Autodesk Fusion 360 part; units mm, degrees
(part 2 of 2)
sketch "スケッチ3" plane through (0, 0, 1.5) normal (0, 0, 1) x (-1, 0, 0)
  line L0 (-5.6421, -16.3724) -> (-10.7928, -25.2936)
  arc A0 (-10.7928, -25.2936) -> (-3.3, -27.3013) centre (0, 0) ccw
  line L1 (-3.3, -27.3013) -> (-3.3, -17)
  line L2 (-3.3, -17) -> (3.3, -17)
  line L3 (3.3, -17) -> (3.3, -27.3013)
  arc A1 (3.3, -27.3013) -> (10.7928, -25.2936) centre (0, 0) ccw
  line L4 (10.7928, -25.2936) -> (5.6421, -16.3724)
  line L5 (5.6421, -16.3724) -> (11.3579, -13.0724)
  line L6 (11.3579, -13.0724) -> (16.5085, -21.9936)
  arc A2 (16.5085, -21.9936) -> (21.9936, -16.5085) centre (0, 0) ccw
  line L7 (21.9936, -16.5085) -> (13.0724, -11.3579)
  line L8 (13.0724, -11.3579) -> (16.3724, -5.6421)
  line L9 (16.3724, -5.6421) -> (25.2936, -10.7928)
  arc A3 (25.2936, -10.7928) -> (27.3013, -3.3) centre (0, 0) ccw
  line L10 (27.3013, -3.3) -> (17, -3.3)
  line L11 (17, -3.3) -> (17, 3.3)
  line L12 (17, 3.3) -> (27.3013, 3.3)
  arc A4 (27.3013, 3.3) -> (25.2936, 10.7928) centre (0, 0) ccw
  line L13 (25.2936, 10.7928) -> (16.3724, 5.6421)
  line L14 (16.3724, 5.6421) -> (13.0724, 11.3579)
  line L15 (13.0724, 11.3579) -> (21.9936, 16.5085)
  arc A5 (21.9936, 16.5085) -> (16.5085, 21.9936) centre (0, 0) ccw
  line L16 (16.5085, 21.9936) -> (11.3579, 13.0724)
  line L17 (11.3579, 13.0724) -> (5.6421, 16.3724)
  line L18 (5.6421, 16.3724) -> (10.7928, 25.2936)
  arc A6 (10.7928, 25.2936) -> (3.3, 27.3013) centre (0, 0) ccw
  line L19 (3.3, 27.3013) -> (3.3, 17)
  line L20 (3.3, 17) -> (-3.3, 17)
  line L21 (-3.3, 17) -> (-3.3, 27.3013)
  arc A7 (-3.3, 27.3013) -> (-10.7928, 25.2936) centre (0, 0) ccw
  line L22 (-10.7928, 25.2936) -> (-5.6421, 16.3724)
  line L23 (-5.6421, 16.3724) -> (-11.3579, 13.0724)
  line L24 (-11.3579, 13.0724) -> (-16.5085, 21.9936)
  arc A8 (-16.5085, 21.9936) -> (-21.9936, 16.5085) centre (0, 0) ccw
  line L25 (-21.9936, 16.5085) -> (-13.0724, 11.3579)
  line L26 (-13.0724, 11.3579) -> (-16.3724, 5.6421)
  line L27 (-16.3724, 5.6421) -> (-25.2936, 10.7928)
  arc A9 (-25.2936, 10.7928) -> (-27.3013, 3.3) centre (0, 0) ccw
  line L28 (-27.3013, 3.3) -> (-17, 3.3)
  line L29 (-17, 3.3) -> (-17, -3.3)
  line L30 (-17, -3.3) -> (-27.3013, -3.3)
  arc A10 (-27.3013, -3.3) -> (-25.2936, -10.7928) centre (0, 0) ccw
  line L31 (-25.2936, -10.7928) -> (-16.3724, -5.6421)
  line L32 (-16.3724, -5.6421) -> (-13.0724, -11.3579)
  line L33 (-13.0724, -11.3579) -> (-21.9936, -16.5085)
  arc A11 (-21.9936, -16.5085) -> (-16.5085, -21.9936) centre (0, 0) ccw
  line L34 (-16.5085, -21.9936) -> (-11.3579, -13.0724)
  line L35 (-11.3579, -13.0724) -> (-5.6421, -16.3724)
  line L36 (3.3, -27.3013) -> (3.3, -26.1013)
  line L37 (3.3, -26.1013) -> (3.3, -23.5013)
  line L38 (3.3, -23.5013) -> (5.3, -23.5013)
  line L39 (5.3, -23.5013) -> (5.3, -26.1013)
  line L40 (5.3, -26.1013) -> (3.3, -26.1013)
  line L41 (3.3, -26.1013) -> (3.3, -23.5013)
  line L42 (-3.3, -27.3013) -> (-3.3, -26.1013)
  line L43 (-3.3, -26.1013) -> (-5.3, -26.1013)
  line L44 (-5.3, -26.1013) -> (-5.3, -23.5013)
  line L45 (-5.3, -23.5013) -> (-3.3, -23.5013)
  line L46 (-3.3, -23.5013) -> (-3.3, -26.1013)
  line L47 (14.6085, -18.7027) -> (16.3406, -17.7027)
  line L48 (16.3406, -17.7027) -> (17.6406, -19.9544)
  line L49 (17.6406, -19.9544) -> (15.9085, -20.9544)
  line L50 (15.9085, -20.9544) -> (14.6085, -18.7027)
  line L51 (8.8928, -22.0027) -> (10.1928, -24.2544)
  line L52 (7.1607, -23.0027) -> (8.8928, -22.0027)
  line L53 (8.4607, -25.2544) -> (7.1607, -23.0027)
  line L54 (10.1928, -24.2544) -> (8.4607, -25.2544)
  line L55 (22.0027, -8.8928) -> (23.0027, -7.1607)
  line L56 (23.0027, -7.1607) -> (25.2544, -8.4607)
  line L57 (25.2544, -8.4607) -> (24.2544, -10.1928)
  line L58 (24.2544, -10.1928) -> (22.0027, -8.8928)
  line L59 (18.7027, -14.6085) -> (20.9544, -15.9085)
  line L60 (17.7027, -16.3406) -> (18.7027, -14.6085)
  line L61 (19.9544, -17.6406) -> (17.7027, -16.3406)
  line L62 (20.9544, -15.9085) -> (19.9544, -17.6406)
  line L63 (23.5013, 3.3) -> (23.5013, 5.3)
  line L64 (23.5013, 5.3) -> (26.1013, 5.3)
  line L65 (26.1013, 5.3) -> (26.1013, 3.3)
  line L66 (26.1013, 3.3) -> (23.5013, 3.3)
  line L67 (23.5013, -3.3) -> (26.1013, -3.3)
  line L68 (23.5013, -5.3) -> (23.5013, -3.3)
  line L69 (26.1013, -5.3) -> (23.5013, -5.3)
  line L70 (26.1013, -3.3) -> (26.1013, -5.3)
  line L71 (18.7027, 14.6085) -> (17.7027, 16.3406)
  line L72 (17.7027, 16.3406) -> (19.9544, 17.6406)
  line L73 (19.9544, 17.6406) -> (20.9544, 15.9085)
  line L74 (20.9544, 15.9085) -> (18.7027, 14.6085)
  line L75 (22.0027, 8.8928) -> (24.2544, 10.1928)
  line L76 (23.0027, 7.1607) -> (22.0027, 8.8928)
  line L77 (25.2544, 8.4607) -> (23.0027, 7.1607)
  line L78 (24.2544, 10.1928) -> (25.2544, 8.4607)
  line L79 (8.8928, 22.0027) -> (7.1607, 23.0027)
  line L80 (7.1607, 23.0027) -> (8.4607, 25.2544)
  line L81 (8.4607, 25.2544) -> (10.1928, 24.2544)
  line L82 (10.1928, 24.2544) -> (8.8928, 22.0027)
  line L83 (14.6085, 18.7027) -> (15.9085, 20.9544)
  line L84 (16.3406, 17.7027) -> (14.6085, 18.7027)
  line L85 (17.6406, 19.9544) -> (16.3406, 17.7027)
  line L86 (15.9085, 20.9544) -> (17.6406, 19.9544)
  line L87 (-3.3, 23.5013) -> (-5.3, 23.5013)
  line L88 (-5.3, 23.5013) -> (-5.3, 26.1013)
  line L89 (-5.3, 26.1013) -> (-3.3, 26.1013)
  line L90 (-3.3, 26.1013) -> (-3.3, 23.5013)
  line L91 (3.3, 23.5013) -> (3.3, 26.1013)
  line L92 (5.3, 23.5013) -> (3.3, 23.5013)
  line L93 (5.3, 26.1013) -> (5.3, 23.5013)
  line L94 (3.3, 26.1013) -> (5.3, 26.1013)
  line L95 (-14.6085, 18.7027) -> (-16.3406, 17.7027)
  line L96 (-16.3406, 17.7027) -> (-17.6406, 19.9544)
  line L97 (-17.6406, 19.9544) -> (-15.9085, 20.9544)
  line L98 (-15.9085, 20.9544) -> (-14.6085, 18.7027)
  line L99 (-8.8928, 22.0027) -> (-10.1928, 24.2544)
  line L100 (-7.1607, 23.0027) -> (-8.8928, 22.0027)
  line L101 (-8.4607, 25.2544) -> (-7.1607, 23.0027)
  line L102 (-10.1928, 24.2544) -> (-8.4607, 25.2544)
  line L103 (-22.0027, 8.8928) -> (-23.0027, 7.1607)
  line L104 (-23.0027, 7.1607) -> (-25.2544, 8.4607)
  line L105 (-25.2544, 8.4607) -> (-24.2544, 10.1928)
  line L106 (-24.2544, 10.1928) -> (-22.0027, 8.8928)
  line L107 (-18.7027, 14.6085) -> (-20.9544, 15.9085)
  line L108 (-17.7027, 16.3406) -> (-18.7027, 14.6085)
  line L109 (-19.9544, 17.6406) -> (-17.7027, 16.3406)
  line L110 (-20.9544, 15.9085) -> (-19.9544, 17.6406)
  line L111 (-23.5013, -3.3) -> (-23.5013, -5.3)
  line L112 (-23.5013, -5.3) -> (-26.1013, -5.3)
  line L113 (-26.1013, -5.3) -> (-26.1013, -3.3)
  line L114 (-26.1013, -3.3) -> (-23.5013, -3.3)
  line L115 (-23.5013, 3.3) -> (-26.1013, 3.3)
  line L116 (-23.5013, 5.3) -> (-23.5013, 3.3)
  line L117 (-26.1013, 5.3) -> (-23.5013, 5.3)
  line L118 (-26.1013, 3.3) -> (-26.1013, 5.3)
  line L119 (-18.7027, -14.6085) -> (-17.7027, -16.3406)
  line L120 (-17.7027, -16.3406) -> (-19.9544, -17.6406)
  line L121 (-19.9544, -17.6406) -> (-20.9544, -15.9085)
  line L122 (-20.9544, -15.9085) -> (-18.7027, -14.6085)
  line L123 (-22.0027, -8.8928) -> (-24.2544, -10.1928)
  line L124 (-23.0027, -7.1607) -> (-22.0027, -8.8928)
  line L125 (-25.2544, -8.4607) -> (-23.0027, -7.1607)
  line L126 (-24.2544, -10.1928) -> (-25.2544, -8.4607)
  line L127 (-8.8928, -22.0027) -> (-7.1607, -23.0027)
  line L128 (-7.1607, -23.0027) -> (-8.4607, -25.2544)
  line L129 (-8.4607, -25.2544) -> (-10.1928, -24.2544)
  line L130 (-10.1928, -24.2544) -> (-8.8928, -22.0027)
  line L131 (-14.6085, -18.7027) -> (-15.9085, -20.9544)
  line L132 (-16.3406, -17.7027) -> (-14.6085, -18.7027)
  line L133 (-17.6406, -19.9544) -> (-16.3406, -17.7027)
  line L134 (-15.9085, -20.9544) -> (-17.6406, -19.9544)
  circle A12 centre (0, -6.25) radius 1.65
  circle A13 centre (5.4127, 3.125) radius 1.65
  circle A14 centre (-5.4127, 3.125) radius 1.65
  line L135 (4.752, 5.6303) -> (0, 2.8868)
  line L136 (0, 2.8868) -> (-4.752, 5.6303)
  line L137 (-4.752, 5.6303) -> (-6.2309, 14.1924)
  arc A15 (6.2309, 14.1924) -> (-6.2309, 14.1924) centre (0, 0) ccw
  line L138 (6.2309, 14.1924) -> (4.752, 5.6303)
  circle A16 centre (0, 0) radius 2.1
  arc A17 (15.4284, 1.4885) -> (9.0033, 12.6171) centre (0, 0) ccw
  line L139 (15.4284, 1.4885) -> (7.5798, 4.3762)
  line L140 (7.5798, 4.3762) -> (9.0033, 12.6171)
  line L141 (2.5, -6.9305) -> (2.5, -1.4434)
  line L142 (2.5, -1.4434) -> (7.252, 1.3002)
  line L143 (7.252, 1.3002) -> (15.4065, -1.7001)
  arc A18 (9.1755, -12.4924) -> (15.4065, -1.7001) centre (0, 0) ccw
  line L144 (9.1755, -12.4924) -> (2.5, -6.9305)
  arc A19 (-9.0033, 12.6171) -> (-15.4284, 1.4885) centre (0, 0) ccw
  line L145 (-9.0033, 12.6171) -> (-7.5798, 4.3762)
  line L146 (-7.5798, 4.3762) -> (-15.4284, 1.4885)
  line L147 (-6.4251, -14.1056) -> (0, -8.7524)
  line L148 (0, -8.7524) -> (6.4251, -14.1056)
  arc A20 (-6.4251, -14.1056) -> (6.4251, -14.1056) centre (0, 0) ccw
  line L149 (-2.5, -6.9305) -> (-9.1755, -12.4924)
  arc A21 (-15.4065, -1.7001) -> (-9.1755, -12.4924) centre (0, 0) ccw
  line L150 (-15.4065, -1.7001) -> (-7.252, 1.3002)
  line L151 (-7.252, 1.3002) -> (-2.5, -1.4434)
  line L152 (-2.5, -1.4434) -> (-2.5, -6.9305)
  dimension "d32" = 1.2
  dimension "d33" = 2.6
  dimension "d34" = 2
  dimension "d35" = 2.6
  dimension "d36" = 1.2
  dimension "d37" = 2
  dimension "d38" = 2.6
  dimension "d40" = 360
  constraint coincident L3.end A1.start
  constraint vertical L36
  constraint parallel L3 L37
  constraint horizontal L38
  constraint vertical L39
  constraint horizontal L40
  constraint vertical L41
  constraint coincident A0.end L1.start
  constraint parallel L1 L42
  constraint horizontal L43
  constraint vertical L44
  constraint horizontal L45
  constraint vertical L46
  measures "d32" distance of L3.end L36.end
  measures "d33" distance of L36.end L37.end
  measures "d34" distance of L37.end L38.end
  measures "d35" distance of L37.end L36.end
  measures "d36" distance of A0.end L42.end
  measures "d37" distance of L42.end L43.end
  measures "d38" distance of L42.end L45.end
extrude "押し出し3" add sketch "スケッチ3" along normal blind 0.5 contours L0 A0 L1 L2 L3 A1 L4 L5 L6 A2 L7 L8 L9 A3 L10 L11 L12 A4 L13 L14 L15 A5 L16 L17 L18 A6 L19 L20 L21 A7 L22 L23 L24 A8 L25 L26 L27 A9 L28 L29 L30 A10 L31 L32 L33 A11 L34 L35 L36 L38 L39 L40 L42 L43 L44 L45 L47 L48 L49 L52 L53 L54 L55 L56 L57 L60 L61 L62 L63 L64 L65 L68 L69 L70 L71 L72 L73 L76 L77 L78 L79 L80 L81 L84 L85 L86 L87 L88 L89 L92 L93 L94 L95 L96 L97 L100 L101 L102 L103 L104 L105 L108 L109 L110 L111 L112 L113 L116 L117 L118 L119 L120 L121 L124 L125 L126 L127 L128 L129 L132 L133 L134
extrude "押し出し4" cut 1 faces at (12.6956, -0.3629, 0) along direction (0, 0, 1) blind 0.5
fillet "フィレット1" radius 1.5 10 edges at (-9.1755, 12.4924, 1.25) (0, -2.8868, 1.25) (-2.5, 1.4434, 1.25) (-2.5, 6.9305, 1.25) (0, 8.7524, 1.25) (-6.4251, 14.1056, 1.25) (6.4251, 14.1056, 1.25) (9.1755, 12.4924, 1.25) (2.5, 6.9305, 1.25) (2.5, 1.4434, 1.25)
fillet "フィレット1" radius 1.5 14 edges at (-4.752, -5.6303, 1.25) (-7.5798, -4.3762, 1.25) (-7.252, -1.3002, 1.25) (-15.4284, -1.4885, 1.25) (-15.4065, 1.7001, 1.25) (-6.2309, -14.1924, 1.25) (-9.0033, -12.6171, 1.25) (6.2309, -14.1924, 1.25) (9.0033, -12.6171, 1.25) (4.752, -5.6303, 1.25) (15.4284, -1.4885, 1.25) (7.5798, -4.3762, 1.25) (7.252, -1.3002, 1.25) (15.4065, 1.7001, 1.25)
fillet "フィレット2" radius 0.5 4 edges at (17.7027, 16.3406, 1.75) (19.9544, 17.6406, 1.75) (23.0027, 7.1607, 1.75) (25.2544, 8.4607, 1.75)
fillet "フィレット3" radius 0.5 44 edges at (17.6406, 19.9544, 1.75) (16.3406, 17.7027, 1.75) (8.4607, 25.2544, 1.75) (5.3, 23.5013, 1.75) (7.1607, 23.0027, 1.75) (5.3, 26.1013, 1.75) (-5.3, 23.5013, 1.75) (-5.3, 26.1013, 1.75) (-8.4607, 25.2544, 1.75) (-7.1607, 23.0027, 1.75) (-17.6406, 19.9544, 1.75) (-16.3406, 17.7027, 1.75) (-19.9544, 17.6406, 1.75) (-17.7027, 16.3406, 1.75) (-25.2544, 8.4607, 1.75) (-23.0027, 7.1607, 1.75) (-23.5013, 5.3, 1.75) (-26.1013, 5.3, 1.75) (-26.1013, -5.3, 1.75) (-23.5013, -5.3, 1.75) (-23.0027, -7.1607, 1.75) (-25.2544, -8.4607, 1.75) (-17.7027, -16.3406, 1.75) (-16.3406, -17.7027, 1.75) (-19.9544, -17.6406, 1.75) (-17.6406, -19.9544, 1.75) (-7.1607, -23.0027, 1.75) (-5.3, -23.5013, 1.75) (-5.3, -26.1013, 1.75) (-8.4607, -25.2544, 1.75) (7.1607, -23.0027, 1.75) (5.3, -23.5013, 1.75) (8.4607, -25.2544, 1.75) (5.3, -26.1013, 1.75) (16.3406, -17.7027, 1.75) (17.7027, -16.3406, 1.75) (19.9544, -17.6406, 1.75) (17.6406, -19.9544, 1.75) (23.5013, -5.3, 1.75) (23.0027, -7.1607, 1.75) (25.2544, -8.4607, 1.75) (26.1013, -5.3, 1.75) (26.1013, 5.3, 1.75) (23.5013, 5.3, 1.75)
fillet "フィレット4" radius 1.5 24 edges at (13.0724, 11.3579, 1.25) (11.3579, 13.0724, 1.25) (5.6421, 16.3724, 1.25) (3.3, 17, 1.25) (-3.3, 17, 1.25) (-5.6421, 16.3724, 1.25) (-11.3579, 13.0724, 1.25) (-13.0724, 11.3579, 1.25) (-16.3724, 5.6421, 1.25) (-17, 3.3, 1.25) (-17, -3.3, 1.25) (-16.3724, -5.6421, 1.25) (-13.0724, -11.3579, 1.25) (-11.3579, -13.0724, 1.25) (-5.6421, -16.3724, 1.25) (-3.3, -17, 1.25) (3.3, -17, 1.25) (5.6421, -16.3724, 1.25) (13.0724, -11.3579, 1.25) (11.3579, -13.0724, 1.25) (17, -3.3, 1.25) (16.3724, -5.6421, 1.25) (17, 3.3, 1.25) (16.3724, 5.6421, 1.25)
extrude "押し出し5" add 1 faces at (6.483, -9.7763, 2) along direction (0, 0, 1) blind 2
extrude "押し出し6" cut 1 faces at (6.483, -9.7763, 4) along direction (0, 0, -1) blind 2

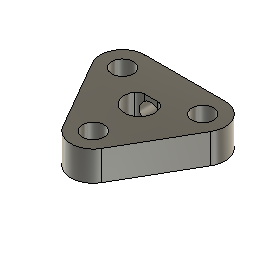
design "オムニ固定"
Autodesk Fusion 360 part; units mm, degrees
sketch "スケッチ1" plane through (0, 0, 0) normal (0, 0, 1) x (1, 0, 0)
  line L0 (2.5981, -7.75) -> (8.0107, 1.625)
  line L1 (0, -6.25) -> (5.4127, 3.125)
  circle A0 centre (5.4127, 3.125) radius 3
  line L2 (5.4127, 3.125) -> (8.0107, 1.625)
  line L3 (5.4127, 3.125) -> (5.4127, 6.125)
  line L4 (5.4127, 3.125) -> (-5.4127, 3.125)
  line L5 (-5.4127, 6.125) -> (5.4127, 6.125)
  circle A1 centre (-5.4127, 3.125) radius 3
  line L6 (-5.4127, 3.125) -> (0, -6.25)
  line L7 (-8.0107, 1.625) -> (-2.5981, -7.75)
  circle A2 centre (0, -6.25) radius 3
  line L8 (0, -6.25) -> (-2.5981, -7.75)
  line L9 (0, -6.25) -> (2.5981, -7.75)
  line L10 (-5.4127, 3.125) -> (-8.0107, 1.625)
  line L11 (-5.4127, 3.125) -> (-5.4127, 6.125)
  circle A3 centre (5.4127, 3.125) radius 1.45
  circle A4 centre (0, 0) radius 2.05
  circle A5 centre (0, -6.25) radius 1.45
  circle A6 centre (-5.4127, 3.125) radius 1.45
  line L12 (0, 0) -> (0, 1.53)
  line L13 (0, 1.53) -> (1.3644, 1.53)
  line L14 (0, 1.53) -> (-1.3644, 1.53)
  dimension "d1" = 6
  dimension "d2" = 6
  dimension "d3" = 6
  dimension "d4" = 2.9
  dimension "d5" = 4.1
  dimension "d6" = 2.9
  dimension "d9" = 2.9
  dimension "d13" = 1.53
  constraint coincident L1.start L6.end
  constraint coincident L1.end A0.centre
  constraint coincident L3.end A0
  constraint vertical L3
  constraint coincident L5.start A1
  constraint perpendicular L4 L11
  constraint coincident L0.end A0
  constraint perpendicular L1 L2
  constraint coincident L0.start A2
  constraint perpendicular L1 L9
  constraint coincident L7.end A2
  constraint perpendicular L6 L8
  constraint coincident L4.end A1.centre
  constraint coincident L7.start A1
  constraint parallel L8 L10
  constraint coincident A4.centre L12.start
  constraint concentric A2 A5
  constraint concentric A1 A6
  constraint vertical L12
  constraint coincident A4 L13.end
  constraint perpendicular L12 L13
  constraint coincident A4 L14.end
  constraint perpendicular L12 L14
  measures "d1" diameter of A2
  measures "d2" diameter of A0
  measures "d3" diameter of A1
  measures "d4" diameter of A3
  measures "d5" diameter of A4
  measures "d6" diameter of A5
  measures "d9" diameter of A6
  measures "d13" distance of A4.centre L12.end
extrude "押し出し1" add sketch "スケッチ1" along normal blind 4 contours L0 L1 A0 A2 | L1 A2 L9 A5 | A2 L8 L9 A5 | A0 L2 L3 A3 | L1 A0 L2 A3 | A1 L6 L7 A2 | L6 A2 L8 A5 | L1 A0 L4 A3 | L1 A0 L4 A1 L6 A2 | A1 L6 L10 A6 | A1 L10 L11 A6 | L1 L6 A2 A5 | A0 L3 L4 A3 | A0 L4 L5 A1 | L4 A1 L11 A6 | L4 A1 L6 A6 | A4 L13 L14 picked at (0.0992, 1.8694)
fillet "フィレット1" radius 0.97 2 edges at (-1.3644, 1.53, 2) (1.3644, 1.53, 2)
sketch "スケッチ2" plane through (0, 6.125, 0) normal (0, 1, 0) x (-1, 0, 0)
  line L0 (-5.4127, 0) -> (5.4127, 0)
  line L1 (5.4127, 0) -> (5.4127, 4)
  line L2 (5.4127, 4) -> (-5.4127, 4)
  line L3 (-5.4127, 4) -> (-5.4127, 0)
  line L4 (-5.4127, 4) -> (5.4127, 0)
  line L5 (-5.4127, 0) -> (5.4127, 4)
  circle A0 centre (0, 2) radius 1.45
  dimension "d16" = 2.9
  constraint coincident L2.end L3.start
  constraint coincident L0.end L1.start
  constraint coincident L0.start L3.end
  constraint coincident L1.end L2.start
  constraint midpoint L4 A0.centre
  measures "d16" diameter of A0
extrude "押し出し2" cut sketch "スケッチ2" against normal blind 7 contours L4 L5 A0 | L4 L5 A0 | L4 L5 A0 | L4 L5 A0

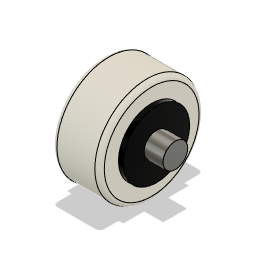
design "サイドホイール v1"
Autodesk Fusion 360 part; units mm, degrees
sketch "スケッチ1" plane through (0, 0, 0) normal (1, 0, 0) x (0, 0, -1)
  circle A0 centre (0, 0) radius 5.5
  circle A1 centre (0, 0) radius 2.5
  circle A2 centre (0, 0) radius 1.3
  circle A3 centre (0, 0) radius 3.5
  dimension "d1" = 11
  dimension "d2" = 5
  dimension "d7" = 2.6
  dimension "d14" = 7
  constraint coincident A0.centre A1.centre
  constraint concentric A0 A1
  constraint concentric A0 A2
  measures "d1" diameter of A0
  measures "d2" diameter of A1
  measures "d7" diameter of A2
  measures "d14" diameter of A3
extrude "押し出し1" add sketch "スケッチ1" along normal blind 5 contours A0 | A3 makes body 1
extrude "押し出し2" add sketch "スケッチ1" along normal blind 5 separate body contours A1 | A2 makes body 2
extrude "押し出し3" cut sketch "スケッチ1" along normal blind 16 contours A2 bodies 2
extrude "押し出し5" add sketch "スケッチ1" against normal blind 0.5 separate body contours A1 | A3 makes body 3
copy_body "ボディのコピーと貼り付け1" bodies 3 makes body 4
move_body "移動1" bodies 4 to x (1, 0, 0) y (0, 1, 0) z (0, 0, 1) at (5.5, 0, 0)
extrude "押し出し6" add sketch "スケッチ1" against normal blind 2.5 separate body contours A2 makes body 5
move_face "面をオフセット1" offset 7.5 1 faces at (0, 0.9052, 0.1692) on bodies 5
fillet "フィレット1" radius 0.5 1 edges at (0, -1.9889, 5.1278) on bodies 1
fillet "フィレット2" radius 0.5 1 edges at (5, -1.9889, 5.1278) on bodies 1
